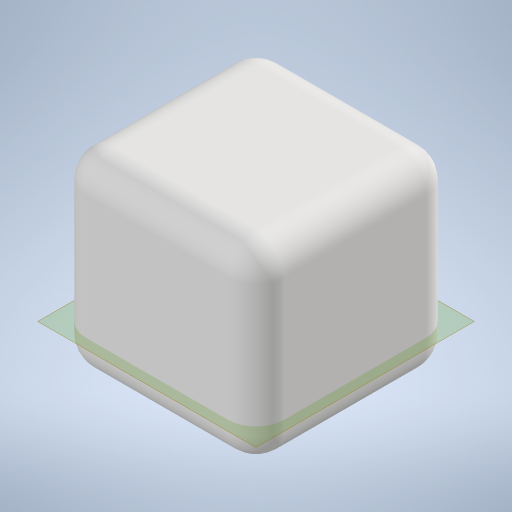
# Autodesk Inventor part: cube
Saved by Autodesk Inventor 2023 (Build 270158000, 158)
## iProperties
Created: 2026-03-04
Part Number: cube
Material: Типовые
Document SubType Name: Modeling
Designer: garin
Density: 1 g/cm^3
Appearance: По умолчанию
Author: garin
Autodesk Inventor part; units mm, degrees
ref_plane "YZ Plane" through (0, 0, 0) normal (1, 0, 0) x (0, 1, 0)
ref_plane "XZ Plane" through (0, 0, 0) normal (0, 1, 0) x (-1, 0, 0)
ref_plane "XY Plane" through (0, 0, 0) normal (0, 0, 1) x (1, 0, 0)
sketch "Эскиз1" plane through (0, 0, 0) normal (0, 1, 0) x (-1, 0, 0)
  line L0 (5.25, 5.25) -> (-5.25, 5.25)
  line L1 (-5.25, 5.25) -> (-5.25, -5.25)
  line L2 (-5.25, -5.25) -> (5.25, -5.25)
  line L3 (5.25, -5.25) -> (5.25, 5.25)
  line L4 (5.25, 0) -> (-5.25, 0) construction
  line L5 (0, 5.25) -> (0, -5.25) construction
  line L6 (3.5, -3.5) -> (-3.5, -3.5)
  line L7 (-3.5, -3.5) -> (-3.5, 3.5)
  line L8 (-3.5, 3.5) -> (3.5, 3.5)
  line L9 (3.5, 3.5) -> (3.5, -3.5)
  line L10 (0, -3.5) -> (0, 3.5) construction
  line L11 (3.5, 0) -> (-3.5, 0) construction
  point P0 (0, 0)
  point P1 (0, 0)
  point P2 (0, 0)
  dimension "d0" = 10.5
  dimension "d1" = 10.5
  dimension "d4" = 7
  dimension "d5" = 7
  constraints: 24 end point, 11 midpoint, 4 parallel, 2 horizontal, 2 perpendicular, 1 coincident
  measures "d0" distance of L2.end L1.end
  measures "d1" distance of L1.end L0.end
  measures "d4" distance of L7.end L8.end
  measures "d5" distance of L6.end L7.end
extrude "Выдавливание1" add sketch "Эскиз1" along normal blind 10 contours L3 L2 L1 L0 | L6 L7 L8 L9
ref_plane "РабПлоскость1" through (0, 2, 0) normal (0, -1, 0) x (1, 0, 0)
extrude "Выдавливание2" cut sketch "Эскиз1" along normal blind 6 from surface at 2 contours L6 L7 L8 L9
fillet "Сопряжение1" radius 1.5 12 edges at (-5.25, 5, -5.25) (-5.25, 0, 0) (0, 0, -5.25) (-5.25, 5, 5.25) (-5.25, 10, 0) (0, 10, -5.25) (0, 10, 5.25) (5.25, 0, 0) (5.25, 5, 5.25) (5.25, 10, 0) (5.25, 5, -5.25) (0, 0, 5.25)
